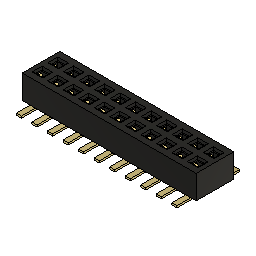
BD050-22-A-0-0500 (Autodesk Fusion 360 design; units mm, degrees)
Autodesk Fusion 360 part; units mm, degrees
note: some values were not read from the file. Chosen so that the rebuilt part matches the saved one: which bodies a step acts on. Set by a fixed rule: which sketch regions a step uses.
(part 1 of 3)
sketch "Sketch5" plane through (0, 0, 0) normal (0, 0, 1) x (1, 0, 0)
  line L0 (28.1987, -12.5621) -> (28.6114, -12.1494)
  line L1 (27.0768, -12.5992) -> (27.3573, -12.3134)
  line L2 (26.7911, -12.5198) -> (27.0768, -12.234)
  line L3 (27.4684, -11.853) -> (27.9817, -11.853)
  line L4 (27.3573, -11.9589) -> (28.1987, -11.9589)
  line L5 (26.68, -11.906) -> (26.8334, -11.7525)
  line L6 (26.8334, -11.7525) -> (26.68, -11.853)
  line L7 (26.68, -11.853) -> (26.68, -11.9589)
  line L8 (27.0768, -12.234) -> (27.4631, -11.8478)
  line L9 (27.0768, -11.8742) -> (27.1985, -11.7525)
  line L10 (27.4684, -11.9589) -> (27.4684, -11.853)
  line L11 (27.4684, -11.853) -> (27.315, -11.7525)
  line L12 (26.7911, -12.1547) -> (27.0768, -11.8742)
  line L13 (28.1987, -12.2023) -> (28.6114, -11.7843)
  line L14 (27.9817, -11.853) -> (27.9817, -11.9589)
  line L15 (28.077, -11.9589) -> (28.2833, -11.7525)
  line L16 (27.9817, -11.853) -> (28.1352, -11.7525)
  line L17 (25.537, -12.6838) -> (25.955, -12.2711)
  line L18 (25.537, -11.9589) -> (25.7486, -11.7525)
  line L19 (25.537, -12.324) -> (26.0714, -11.7895)
  line L20 (26.1667, -11.9589) -> (26.1667, -11.853)
  line L21 (26.1667, -11.853) -> (26.0132, -11.7525)
  line L22 (25.537, -11.7525) -> (28.6114, -11.7525)
  line L23 (26.7911, -11.9589) -> (25.955, -11.9589)
  line L24 (26.68, -11.853) -> (26.1667, -11.853)
  line L25 (27.0768, -13.684) -> (27.3573, -13.4035)
  line L26 (26.7911, -13.6046) -> (27.0768, -13.3241)
  line L27 (27.061, -13.6998) -> (27.0768, -13.684)
  line L28 (27.0768, -13.3241) -> (27.3573, -13.0384)
  line L29 (26.7911, -13.2395) -> (27.0768, -12.959)
  line L30 (28.1987, -13.6469) -> (28.6114, -13.2342)
  line L31 (28.6114, -13.8004) -> (28.3098, -13.8004)
  line L32 (28.3098, -13.8004) -> (28.1987, -13.6998)
  line L33 (28.405, -13.8004) -> (28.6114, -13.594)
  line L34 (28.1987, -13.2871) -> (28.6114, -12.8743)
  line L35 (25.537, -13.4088) -> (25.955, -12.996)
  line L36 (25.537, -13.7739) -> (25.955, -13.3559)
  line L37 (25.537, -13.8004) -> (25.8386, -13.8004)
  line L38 (25.8386, -13.8004) -> (25.955, -13.6998)
  line L39 (25.955, -13.6998) -> (28.1987, -13.6998)
  line L40 (28.1987, -13.6998) -> (28.1987, -11.9589)
  line L41 (28.6114, -11.7525) -> (28.6114, -13.8004)
  line L42 (27.3573, -11.9589) -> (27.3573, -13.6998)
  line L43 (26.7911, -11.9589) -> (26.7911, -13.6998)
  line L44 (25.955, -11.9589) -> (25.955, -13.6998)
  line L45 (27.8759, -12.16) -> (27.8706, -12.1335)
  line L46 (27.8706, -12.1335) -> (27.86, -12.107)
  line L47 (27.86, -12.107) -> (27.8441, -12.0912)
  line L48 (27.8441, -12.0912) -> (27.823, -12.0753)
  line L49 (27.823, -12.0753) -> (27.8018, -12.0647)
  line L50 (27.8018, -12.0647) -> (27.7753, -12.0594)
  line L51 (27.7753, -12.0594) -> (27.5795, -12.0594)
  line L52 (27.5795, -12.0594) -> (27.5531, -12.0647)
  line L53 (27.5531, -12.0647) -> (27.5266, -12.0753)
  line L54 (27.5266, -12.0753) -> (27.4949, -12.107)
  line L55 (27.4949, -12.107) -> (27.4843, -12.1335)
  line L56 (27.4843, -12.1335) -> (27.479, -12.16)
  line L57 (27.479, -12.16) -> (27.479, -13.086)
  line L58 (27.479, -13.086) -> (27.3255, -13.2871)
  line L59 (27.3255, -13.2871) -> (27.389, -13.2871)
  line L60 (27.4472, -13.3506) -> (27.442, -13.3294)
  line L61 (27.442, -13.3294) -> (27.4314, -13.3082)
  line L62 (27.4314, -13.3082) -> (27.4102, -13.2977)
  line L63 (27.4102, -13.2977) -> (27.389, -13.2924)
  line L64 (27.4472, -13.3506) -> (27.4472, -13.4935)
  line L65 (27.4525, -13.4935) -> (27.4578, -13.5199)
  line L66 (27.4578, -13.5199) -> (27.4684, -13.5411)
  line L67 (27.4684, -13.5411) -> (27.4843, -13.5623)
  line L68 (27.4843, -13.5623) -> (27.5002, -13.5781)
  line L69 (27.5002, -13.5781) -> (27.5266, -13.5887)
  line L70 (27.5266, -13.5887) -> (27.5531, -13.594)
  line L71 (27.5531, -13.594) -> (28.0452, -13.594)
  line L72 (28.0452, -13.594) -> (28.0452, -13.721)
  line L73 (28.0452, -13.721) -> (28.0505, -13.7686)
  line L74 (28.0505, -13.7686) -> (28.0611, -13.811)
  line L75 (28.0611, -13.811) -> (28.0822, -13.848)
  line L76 (28.0822, -13.848) -> (28.114, -13.885)
  line L77 (28.114, -13.885) -> (28.151, -13.9168)
  line L78 (28.151, -13.9168) -> (28.1881, -13.938)
  line L79 (28.1881, -13.938) -> (28.2304, -13.9485)
  line L80 (28.2304, -13.9485) -> (28.278, -13.9538)
  line L81 (28.278, -13.9538) -> (29.638, -13.9538)
  line L82 (29.638, -13.9538) -> (29.638, -13.8004)
  line L83 (29.638, -13.8004) -> (28.278, -13.8004)
  line L84 (28.1987, -13.721) -> (28.204, -13.7422)
  line L85 (28.204, -13.7422) -> (28.2092, -13.758)
  line L86 (28.2092, -13.758) -> (28.2198, -13.7792)
  line L87 (28.2198, -13.7792) -> (28.2357, -13.7898)
  line L88 (28.2357, -13.7898) -> (28.278, -13.8004)
  line L89 (28.1987, -13.721) -> (28.1987, -12.8796)
  line L90 (28.1987, -12.8796) -> (27.9817, -12.8796)
  line L91 (27.8812, -12.7738) -> (27.8865, -12.8002)
  line L92 (27.8865, -12.8002) -> (27.897, -12.8214)
  line L93 (27.897, -12.8214) -> (27.9129, -12.8426)
  line L94 (27.9129, -12.8426) -> (27.9288, -12.8585)
  line L95 (27.9288, -12.8585) -> (27.9552, -12.869)
  line L96 (27.9552, -12.869) -> (27.9817, -12.8743)
  line L97 (27.8812, -12.7738) -> (27.8812, -12.16)
  line L98 (25.537, -11.7525) -> (25.537, -13.8004)
  line L99 (26.373, -12.0594) -> (26.3466, -12.0647)
  line L100 (26.3466, -12.0647) -> (26.3201, -12.0753)
  line L101 (26.3201, -12.0753) -> (26.2884, -12.107)
  line L102 (26.2884, -12.107) -> (26.2778, -12.1335)
  line L103 (26.2778, -12.1335) -> (26.2725, -12.16)
  line L104 (26.373, -12.0594) -> (26.5688, -12.0594)
  line L105 (26.6694, -12.16) -> (26.6641, -12.1335)
  line L106 (26.6641, -12.1335) -> (26.6535, -12.107)
  line L107 (26.6535, -12.107) -> (26.6376, -12.0912)
  line L108 (26.6376, -12.0912) -> (26.6165, -12.0753)
  line L109 (26.6165, -12.0753) -> (26.5953, -12.0647)
  line L110 (26.5953, -12.0647) -> (26.5688, -12.0594)
  line L111 (26.6694, -12.16) -> (26.6694, -13.086)
  line L112 (26.6694, -13.086) -> (26.8281, -13.2871)
  line L113 (26.8281, -13.2871) -> (26.7646, -13.2871)
  line L114 (26.7646, -13.2924) -> (26.7435, -13.2977)
  line L115 (26.7435, -13.2977) -> (26.7223, -13.3083)
  line L116 (26.7223, -13.3083) -> (26.7117, -13.3294)
  line L117 (26.7117, -13.3294) -> (26.7064, -13.3506)
  line L118 (26.7011, -13.3506) -> (26.7011, -13.4935)
  line L119 (26.6006, -13.594) -> (26.627, -13.5887)
  line L120 (26.627, -13.5887) -> (26.6535, -13.5781)
  line L121 (26.6535, -13.5781) -> (26.6694, -13.5622)
  line L122 (26.6694, -13.5622) -> (26.6852, -13.5411)
  line L123 (26.6852, -13.5411) -> (26.6958, -13.5199)
  line L124 (26.6958, -13.5199) -> (26.7011, -13.4935)
  line L125 (26.6006, -13.594) -> (26.1085, -13.594)
  line L126 (26.1085, -13.594) -> (26.1085, -13.721)
  line L127 (25.8703, -13.9538) -> (25.918, -13.9485)
  line L128 (25.918, -13.9485) -> (25.9603, -13.938)
  line L129 (25.9603, -13.938) -> (25.9973, -13.9168)
  line L130 (25.9973, -13.9168) -> (26.0344, -13.885)
  line L131 (26.0344, -13.885) -> (26.0661, -13.848)
  line L132 (26.0661, -13.848) -> (26.0873, -13.811)
  line L133 (26.0873, -13.811) -> (26.0979, -13.7686)
  line L134 (26.0979, -13.7686) -> (26.1032, -13.721)
  line L135 (25.8703, -13.9538) -> (24.5104, -13.9538)
  line L136 (24.5104, -13.9538) -> (24.5104, -13.8004)
  line L137 (24.5104, -13.8004) -> (25.8703, -13.8004)
  line L138 (25.8703, -13.8004) -> (25.8915, -13.7951)
  line L139 (25.8915, -13.7951) -> (25.9074, -13.7898)
  line L140 (25.9074, -13.7898) -> (25.9285, -13.7792)
  line L141 (25.9285, -13.7792) -> (25.9391, -13.758)
  line L142 (25.9391, -13.758) -> (25.9444, -13.7422)
  line L143 (25.9444, -13.7422) -> (25.9497, -13.721)
  line L144 (25.955, -13.721) -> (25.955, -12.8796)
  line L145 (25.955, -12.8796) -> (26.1667, -12.8796)
  line L146 (26.1667, -12.8743) -> (26.1931, -12.869)
  line L147 (26.1931, -12.869) -> (26.2143, -12.8585)
  line L148 (26.2143, -12.8585) -> (26.2355, -12.8426)
  line L149 (26.2355, -12.8426) -> (26.2513, -12.8267)
  line L150 (26.2513, -12.8267) -> (26.2619, -12.8002)
  line L151 (26.2619, -12.8002) -> (26.2672, -12.7738)
  line L152 (26.2725, -12.7738) -> (26.2725, -12.16)
  line L153 (27.0768, -11.4615) -> (27.0768, -12.832)
  line L154 (27.0768, -13.086) -> (27.0768, -13.3453)
  line L155 (27.0768, -13.5993) -> (27.0768, -14.9698)
  line L156 (25.537, -13.049) -> (25.955, -12.6309)
  line L157 (27.0768, -12.959) -> (27.3573, -12.6785)
  line L158 (26.7911, -12.8796) -> (27.0768, -12.5992)
  line L159 (28.1987, -12.9272) -> (28.6114, -12.5092)
  line L160 (13.165, 1.9) -> (12.8581, 1.9)
  line L161 (14.4668, 1.9) -> (14.1599, 1.9)
  line L162 (14.5991, -0.296) -> (14.5991, 0.2702)
  line L163 (14.5991, 0.2702) -> (14.7261, 0.3972)
  line L164 (12.7311, 0.2702) -> (12.7311, -0.296)
  line L165 (11.9956, 0.2702) -> (11.9956, -0.296)
  line L166 (13.2973, 0.2702) -> (13.2973, -0.296)
  line L167 (13.2973, -0.296) -> (12.7311, -0.296)
  line L168 (11.9956, 0.2702) -> (12.1226, 0.3972)
  line L169 (13.4243, 0.3972) -> (13.2973, 0.2702)
  line L170 (13.2973, 0.2702) -> (12.7311, 0.2702)
  line L171 (12.7311, 0.2702) -> (12.6041, 0.3972)
  line L172 (12.6041, 0.3972) -> (13.4243, 0.3972)
  line L173 (14.0329, -0.296) -> (14.0329, 0.2702)
  line L174 (14.0329, 0.2702) -> (13.9059, 0.3972)
  line L175 (14.5991, -0.296) -> (14.0329, -0.296)
  line L176 (14.7261, 0.3972) -> (13.9059, 0.3972)
  line L177 (14.5991, 0.2702) -> (14.0329, 0.2702)
  line L178 (11.8686, 0.8734) -> (11.8686, 1.9)
  line L179 (13.165, 0.8734) -> (13.165, 1.9)
  line L180 (12.8581, 0.8734) -> (12.8581, 1.9)
  line L181 (14.4668, 0.8734) -> (14.4668, 1.9)
  line L182 (14.1599, 0.8734) -> (14.1599, 1.9)
  line L183 (10.5668, 1.9) -> (10.2546, 1.9)
  line L184 (7.9633, 1.9) -> (7.6564, 1.9)
  line L185 (7.6564, 1.9) -> (7.6564, 0.8734)
  line L186 (7.9633, 0.8734) -> (7.9633, 1.9)
  line L187 (9.2651, 0.8734) -> (9.2651, 1.9)
  line L188 (8.9582, 0.8734) -> (8.9582, 1.9)
  line L189 (8.9582, 1.9) -> (9.2651, 1.9)
  line L190 (10.6938, 0.2702) -> (10.6938, -0.296)
  line L191 (10.1276, 0.2702) -> (10.1276, -0.296)
  line L192 (11.4294, 0.2702) -> (11.4294, -0.296)
  line L193 (10.6938, -0.296) -> (10.1276, -0.296)
  line L194 (10.1276, 0.2702) -> (10.0006, 0.3972)
  line L195 (10.0006, 0.3972) -> (10.8208, 0.3972)
  line L196 (10.8208, 0.3972) -> (10.6938, 0.2702)
  line L197 (10.6938, 0.2702) -> (10.1276, 0.2702)
  line L198 (11.4294, 0.2702) -> (11.3024, 0.3972)
  line L199 (10.2546, 0.8734) -> (10.2546, 1.9)
  line L200 (10.5668, 0.8734) -> (10.5668, 1.9)
  line L201 (11.5564, 0.8734) -> (11.5564, 1.9)
  line L202 (-0.8367, 0.8734) -> (15.1494, 0.8734)
  line L203 (11.9956, -0.296) -> (11.4294, -0.296)
  line L204 (11.9956, 0.2702) -> (11.4294, 0.2702)
  line L205 (12.1226, 0.3972) -> (11.3024, 0.3972)
  line L206 (11.8686, 1.9) -> (11.5564, 1.9)
  line L207 (14.5991, -1.0316) -> (14.7261, -0.9046)
  line L208 (11.9956, -1.0316) -> (12.1226, -0.9046)
  line L209 (12.7311, -1.0316) -> (13.2973, -1.0316)
  line L210 (13.2973, -1.0316) -> (13.4243, -0.9046)
  line L211 (13.4243, -0.9046) -> (12.6041, -0.9046)
  line L212 (13.4243, -0.423) -> (12.6041, -0.423)
  line L213 (12.7311, -1.0316) -> (12.6041, -0.9046)
  line L214 (14.0329, -1.0316) -> (13.9059, -0.9046)
  line L215 (13.9059, -0.9046) -> (14.7261, -0.9046)
  line L216 (14.7261, -0.423) -> (13.9059, -0.423)
  line L217 (14.5991, -1.0316) -> (14.0329, -1.0316)
  line L218 (14.5991, -1.5978) -> (14.7261, -1.7248)
  line L219 (11.9956, -1.5978) -> (12.1226, -1.7248)
  line L220 (12.7311, -1.5978) -> (13.2973, -1.5978)
  line L221 (13.2973, -1.5978) -> (13.4243, -1.7248)
  line L222 (13.4243, -1.7248) -> (12.6041, -1.7248)
  line L223 (12.6041, -1.7248) -> (12.7311, -1.5978)
  line L224 (14.0329, -1.5978) -> (13.9059, -1.7248)
  line L225 (13.9059, -1.7248) -> (14.7261, -1.7248)
  line L226 (14.5991, -1.5978) -> (14.0329, -1.5978)
  line L227 (13.2973, -1.5978) -> (13.2973, -1.0316)
  line L228 (13.4243, -1.7248) -> (13.4243, -0.9046)
  line L229 (12.6041, -1.7248) -> (12.6041, -0.9046)
  line L230 (11.9956, -1.5978) -> (11.9956, -1.0316)
  line L231 (12.1226, -1.7248) -> (12.1226, -0.9046)
  line L232 (12.7311, -1.5978) -> (12.7311, -1.0316)
  line L233 (14.5991, -1.5978) -> (14.5991, -1.0316)
  line L234 (14.0329, -1.5978) -> (14.0329, -1.0316)
  line L235 (13.9059, -1.7248) -> (13.9059, -0.9046)
  line L236 (14.7261, -1.7248) -> (14.7261, -0.9046)
  line L237 (10.1276, -1.0316) -> (10.0006, -0.9046)
  line L238 (10.0006, -0.9046) -> (10.8208, -0.9046)
  line L239 (10.8208, -0.423) -> (10.0006, -0.423)
  line L240 (10.8208, -0.9046) -> (10.6938, -1.0316)
  line L241 (10.6938, -1.0316) -> (10.1276, -1.0316)
  line L242 (11.4294, -1.0316) -> (11.3024, -0.9046)
  line L243 (10.1276, -1.5978) -> (10.0006, -1.7248)
  line L244 (10.0006, -1.7248) -> (10.8208, -1.7248)
  line L245 (10.8208, -1.7248) -> (10.6938, -1.5978)
  line L246 (10.6938, -1.5978) -> (10.1276, -1.5978)
  line L247 (11.4294, -1.5978) -> (11.3024, -1.7248)
  line L248 (10.6938, -1.5978) -> (10.6938, -1.0316)
  line L249 (10.8208, -1.7248) -> (10.8208, -0.9046)
  line L250 (10.1276, -1.5978) -> (10.1276, -1.0316)
  line L251 (10.0006, -1.7248) -> (10.0006, -0.9046)
  line L252 (11.4294, -1.5978) -> (11.4294, -1.0316)
  line L253 (11.3024, -1.7248) -> (11.3024, -0.9046)
  line L254 (-0.8367, -2.201) -> (15.1494, -2.201)
  line L255 (11.9956, -1.5978) -> (11.4294, -1.5978)
  line L256 (12.1226, -1.7248) -> (11.3024, -1.7248)
  line L257 (11.9956, -1.0316) -> (11.4294, -1.0316)
  line L258 (12.1226, -0.9046) -> (11.3024, -0.9046)
  line L259 (12.1226, -0.423) -> (11.3024, -0.423)
  line L260 (10.8208, 0.3972) -> (10.8208, -0.423)
  line L261 (10.0006, 0.3972) -> (10.0006, -0.423)
  line L262 (11.3024, 0.3972) -> (11.3024, -0.423)
  line L263 (12.6041, 0.3972) -> (12.6041, -0.423)
  line L264 (12.1226, 0.3972) -> (12.1226, -0.423)
  line L265 (13.4243, 0.3972) -> (13.4243, -0.423)
  line L266 (10.1276, -0.296) -> (10.0006, -0.423)
  line L267 (10.6938, -0.296) -> (10.8208, -0.423)
  line L268 (11.9956, -0.296) -> (12.1226, -0.423)
  line L269 (11.4294, -0.296) -> (11.3024, -0.423)
  line L270 (13.2973, -0.296) -> (13.4243, -0.423)
  line L271 (12.7311, -0.296) -> (12.6041, -0.423)
  line L272 (13.9059, 0.3972) -> (13.9059, -0.423)
  line L273 (15.1494, -2.201) -> (15.1494, 0.8734)
  line L274 (15.1494, 0.8734) -> (15.1494, -2.201)
  line L275 (14.7261, 0.3972) -> (14.7261, -0.423)
  line L276 (14.7261, -0.423) -> (14.5991, -0.296)
  line L277 (14.0329, -0.296) -> (13.9059, -0.423)
  line L278 (6.6616, 1.9) -> (6.3547, 1.9)
  line L279 (5.0529, 1.9) -> (5.3598, 1.9)
  line L280 (5.3598, 1.9) -> (5.3598, 0.8734)
  line L281 (5.0529, 0.8734) -> (5.0529, 1.9)
  line L282 (6.3547, 0.8734) -> (6.3547, 1.9)
  line L283 (6.6616, 0.8734) -> (6.6616, 1.9)
  line L284 (2.7563, 1.9) -> (2.4494, 1.9)
  line L285 (4.0581, 1.9) -> (3.7512, 1.9)
  line L286 (3.4919, 0.3972) -> (4.3121, 0.3972)
  line L287 (4.3121, 0.3972) -> (4.1851, 0.2702)
  line L288 (2.8833, 0.2702) -> (2.8833, -0.296)
  line L289 (2.3224, 0.2702) -> (2.3224, -0.296)
  line L290 (3.6242, 0.2702) -> (3.6242, -0.296)
  line L291 (4.1851, 0.2702) -> (4.1851, -0.296)
  line L292 (2.3224, -0.296) -> (2.8833, -0.296)
  line L293 (3.6242, -0.296) -> (4.1851, -0.296)
  line L294 (2.8833, 0.2702) -> (3.0103, 0.3972)
  line L295 (2.1901, 0.3972) -> (2.3224, 0.2702)
  line L296 (2.3224, 0.2702) -> (2.8833, 0.2702)
  line L297 (2.1901, 0.3972) -> (3.0103, 0.3972)
  line L298 (3.4919, 0.3972) -> (3.6242, 0.2702)
  line L299 (3.6242, 0.2702) -> (4.1851, 0.2702)
  line L300 (2.7563, 0.8734) -> (2.7563, 1.9)
  line L301 (2.4494, 0.8734) -> (2.4494, 1.9)
  line L302 (3.7512, 0.8734) -> (3.7512, 1.9)
  line L303 (4.0581, 0.8734) -> (4.0581, 1.9)
  line L304 (0.1528, 1.9) -> (-0.1541, 1.9)
  line L305 (1.4546, 1.9) -> (1.1477, 1.9)
  line L306 (1.5816, 0.2702) -> (1.5816, -0.296)
  line L307 (0.2798, 0.2702) -> (0.2798, -0.296)
  line L308 (1.0207, 0.2702) -> (1.0207, -0.296)
  line L309 (1.0207, -0.296) -> (1.5816, -0.296)
  line L310 (0.2798, 0.2702) -> (0.4121, 0.3972)
  line L311 (1.7086, 0.3972) -> (1.5816, 0.2702)
  line L312 (1.5816, 0.2702) -> (1.0207, 0.2702)
  line L313 (1.0207, 0.2702) -> (0.8937, 0.3972)
  line L314 (0.8937, 0.3972) -> (1.7086, 0.3972)
  line L315 (-0.2811, -0.296) -> (-0.2811, 0.2702)
  line L316 (-0.2811, 0.2702) -> (-0.4081, 0.3972)
  line L317 (-0.2811, -0.296) -> (0.2798, -0.296)
  line L318 (-0.4081, 0.3972) -> (0.4121, 0.3972)
  line L319 (-0.2811, 0.2702) -> (0.2798, 0.2702)
  line L320 (1.4546, 0.8734) -> (1.4546, 1.9)
  line L321 (0.1528, 0.8734) -> (0.1528, 1.9)
  line L322 (-0.1541, 0.8734) -> (-0.1541, 1.9)
  line L323 (1.1477, 0.8734) -> (1.1477, 1.9)
  line L324 (3.4919, -0.9046) -> (4.3121, -0.9046)
  line L325 (3.4919, -0.423) -> (4.3121, -0.423)
  line L326 (4.1851, -1.0316) -> (4.3121, -0.9046)
  line L327 (2.8833, -1.0316) -> (3.0103, -0.9046)
  line L328 (2.3224, -1.0316) -> (2.1901, -0.9046)
  line L329 (2.1901, -0.9046) -> (3.0103, -0.9046)
  line L330 (2.3224, -1.0316) -> (2.8833, -1.0316)
  line L331 (2.1901, -0.423) -> (3.0103, -0.423)
  line L332 (3.4919, -0.9046) -> (3.6242, -1.0316)
  line L333 (3.6242, -1.0316) -> (4.1851, -1.0316)
  line L334 (3.4919, -1.7248) -> (4.3121, -1.7248)
  line L335 (4.3121, -1.7248) -> (4.1851, -1.5978)
  line L336 (2.8833, -1.5978) -> (3.0103, -1.7248)
  line L337 (2.3224, -1.5978) -> (2.1901, -1.7248)
  line L338 (2.1901, -1.7248) -> (3.0103, -1.7248)
  line L339 (2.3224, -1.5978) -> (2.8833, -1.5978)
  line L340 (3.4919, -1.7248) -> (3.6242, -1.5978)
  line L341 (3.6242, -1.5978) -> (4.1851, -1.5978)
  line L342 (3.4919, -1.7248) -> (3.4919, -0.9046)
  line L343 (3.6242, -1.5978) -> (3.6242, -1.0316)
  line L344 (3.0103, -1.7248) -> (3.0103, -0.9046)
  line L345 (2.8833, -1.5978) -> (2.8833, -1.0316)
  line L346 (2.1901, -1.7248) -> (2.1901, -0.9046)
  line L347 (2.3224, -1.5978) -> (2.3224, -1.0316)
  line L348 (4.1851, -1.5978) -> (4.1851, -1.0316)
  line L349 (4.3121, -1.7248) -> (4.3121, -0.9046)
  line L350 (0.2798, -1.0316) -> (0.4121, -0.9046)
  line L351 (1.7086, -0.9046) -> (1.5816, -1.0316)
  line L352 (1.5816, -1.0316) -> (1.0207, -1.0316)
  line L353 (0.8937, -0.423) -> (1.7086, -0.423)
  line L354 (1.7086, -0.9046) -> (0.8937, -0.9046)
  line L355 (0.8937, -0.9046) -> (1.0207, -1.0316)
  line L356 (-0.2811, -1.0316) -> (-0.4081, -0.9046)
  line L357 (-0.4081, -0.9046) -> (0.4121, -0.9046)
  line L358 (-0.2811, -1.0316) -> (0.2798, -1.0316)
  line L359 (-0.4081, -0.423) -> (0.4121, -0.423)
  line L360 (0.2798, -1.5978) -> (0.4121, -1.7248)
  line L361 (1.7086, -1.7248) -> (1.5816, -1.5978)
  line L362 (1.5816, -1.5978) -> (1.0207, -1.5978)
  line L363 (1.7086, -1.7248) -> (0.8937, -1.7248)
  line L364 (0.8937, -1.7248) -> (1.0207, -1.5978)
  line L365 (-0.2811, -1.5978) -> (-0.4081, -1.7248)
  line L366 (-0.4081, -1.7248) -> (0.4121, -1.7248)
  line L367 (-0.2811, -1.5978) -> (0.2798, -1.5978)
  line L368 (0.2798, -1.5978) -> (0.2798, -1.0316)
  line L369 (0.4121, -1.7248) -> (0.4121, -0.9046)
  line L370 (1.0207, -1.5978) -> (1.0207, -1.0316)
  line L371 (0.8937, -1.7248) -> (0.8937, -0.9046)
  line L372 (1.7086, -1.7248) -> (1.7086, -0.9046)
  line L373 (1.5816, -1.5978) -> (1.5816, -1.0316)
  line L374 (-0.4081, -1.7248) -> (-0.4081, -0.9046)
  line L375 (-0.2811, -1.5978) -> (-0.2811, -1.0316)
  line L376 (-0.8367, 0.8734) -> (-0.8367, -2.201)
  line L377 (4.1851, -0.296) -> (4.3121, -0.423)
  line L378 (3.4919, 0.3972) -> (3.4919, -0.423)
  line L379 (0.4121, 0.3972) -> (0.4121, -0.423)
  line L380 (0.8937, 0.3972) -> (0.8937, -0.423)
  line L381 (3.0103, 0.3972) -> (3.0103, -0.423)
  line L382 (2.1901, 0.3972) -> (2.1901, -0.423)
  line L383 (1.7086, 0.3972) -> (1.7086, -0.423)
  line L384 (-0.4081, 0.3972) -> (-0.4081, -0.423)
  line L385 (0.2798, -0.296) -> (0.4121, -0.423)
  line L386 (-0.2811, -0.296) -> (-0.4081, -0.423)
  line L387 (1.5816, -0.296) -> (1.7086, -0.423)
  line L388 (1.0207, -0.296) -> (0.8937, -0.423)
  line L389 (2.8833, -0.296) -> (3.0103, -0.423)
  line L390 (2.3224, -0.296) -> (2.1901, -0.423)
  line L391 (3.6242, -0.296) -> (3.4919, -0.423)
  line L392 (4.3121, 0.3972) -> (4.3121, -0.423)
  line L393 (13.165, -3.2276) -> (12.8581, -3.2276)
  line L394 (14.4668, -3.2276) -> (14.1599, -3.2276)
  line L395 (10.5668, -3.2276) -> (10.2546, -3.2276)
  line L396 (7.9633, -3.2276) -> (7.6564, -3.2276)
  line L397 (9.2651, -3.2276) -> (8.9582, -3.2276)
  line L398 (11.8686, -3.2276) -> (11.5564, -3.2276)
  line L399 (14.7261, -11.7525) -> (14.5991, -11.853)
  line L400 (14.5991, -11.853) -> (14.5991, -11.9589)
  line L401 (13.5831, -11.7525) -> (13.6678, -12.287)
  line L402 (13.9059, -11.7525) -> (14.0329, -11.853)
  line L403 (14.0329, -11.853) -> (14.0329, -11.9589)
  line L404 (13.8159, -11.9589) -> (14.8108, -11.9589)
  line L405 (14.0329, -11.853) -> (14.5991, -11.853)
  line L406 (-0.8367, -11.7525) -> (15.1494, -11.7525)
  line L407 (14.5303, -13.594) -> (14.7843, -13.594)
  line L408 (14.5303, -13.8004) -> (15.1494, -13.8004)
  line L409 (14.5303, -13.6998) -> (15.1494, -13.6998)
  line L410 (14.5303, -13.594) -> (14.5303, -13.9538)
  line L411 (14.6308, -13.0331) -> (14.7843, -13.0331)
  line L412 (13.5249, -13.2712) -> (13.6625, -13.8004)
  line L413 (11.9268, -13.9538) -> (11.9268, -13.8004)
  line L414 (12.7999, -13.9538) -> (13.2285, -13.9538)
  line L415 (13.2285, -13.8004) -> (12.7999, -13.8004)
  line L416 (12.7999, -13.8004) -> (12.7999, -13.9538)
  line L417 (13.2285, -13.9538) -> (13.2285, -13.8004)
  line L418 (14.1017, -13.9538) -> (14.1017, -13.594)
  line L419 (14.1017, -13.594) -> (13.8424, -13.594)
  line L420 (13.636, -13.6998) -> (14.1017, -13.6998)
  line L421 (13.8424, -13.0331) -> (13.9958, -13.0331)
  line L422 (14.5303, -13.9538) -> (14.1017, -13.9538)
  line L423 (14.5303, -13.8004) -> (14.1017, -13.8004)
  line L424 (13.9958, -12.8796) -> (14.6308, -12.8796)
  line L425 (10.625, -13.9538) -> (10.625, -13.8004)
  line L426 (10.1964, -13.9538) -> (10.1964, -13.8004)
  line L427 (10.1964, -13.8004) -> (10.625, -13.8004)
  line L428 (10.1964, -13.9538) -> (10.625, -13.9538)
  line L429 (11.4982, -13.8004) -> (11.4982, -13.9538)
  line L430 (8.8947, -13.8004) -> (9.3233, -13.8004)
  line L431 (8.8947, -13.9538) -> (9.3233, -13.9538)
  line L432 (7.5929, -13.8004) -> (8.0215, -13.8004)
  line L433 (8.0215, -13.9538) -> (7.5929, -13.9538)
  line L434 (7.5929, -13.9538) -> (7.5929, -13.8004)
  line L435 (8.8947, -13.8004) -> (8.8947, -13.9538)
  line L436 (8.0215, -13.9538) -> (8.0215, -13.8004)
  line L437 (9.3233, -13.9538) -> (9.3233, -13.8004)
  line L438 (11.4982, -13.9538) -> (11.9268, -13.9538)
  line L439 (11.4982, -13.8004) -> (11.9268, -13.8004)
  line L440 (7.159, -11.3715) -> (7.159, -12.3981)
  line L441 (7.159, -12.6521) -> (7.159, -12.9114)
  line L442 (7.159, -13.1654) -> (7.159, -14.192)
  line L443 (14.7843, -13.594) -> (14.7843, -12.795)
  line L444 (14.7843, -12.795) -> (14.7843, -12.7579)
  line L445 (14.7843, -12.7579) -> (14.7737, -12.7156)
  line L446 (14.779, -12.7209) -> (14.6467, -12.4034)
  line L447 (14.652, -12.3134) -> (14.6467, -12.3346)
  line L448 (14.6467, -12.3346) -> (14.6414, -12.361)
  line L449 (14.6414, -12.361) -> (14.6414, -12.3822)
  line L450 (14.6414, -12.3822) -> (14.6467, -12.4034)
  line L451 (14.652, -12.3134) -> (14.7367, -12.1123)
  line L452 (14.7367, -12.1123) -> (14.5938, -12.0594)
  line L453 (14.5938, -12.0594) -> (14.5091, -12.2605)
  line L454 (14.5038, -12.2605) -> (14.4933, -12.3081)
  line L455 (14.4933, -12.3081) -> (14.488, -12.3505)
  line L456 (14.488, -12.3505) -> (14.488, -12.3981)
  line L457 (14.488, -12.3981) -> (14.4985, -12.4457)
  line L458 (14.4985, -12.4457) -> (14.6255, -12.7579)
  line L459 (14.6308, -12.795) -> (14.6308, -12.7738)
  line L460 (14.6308, -12.7738) -> (14.6255, -12.7579)
  line L461 (14.6308, -12.795) -> (14.6308, -13.594)
  line L462 (13.8424, -13.594) -> (13.8424, -12.795)
  line L463 (13.853, -12.7156) -> (13.8424, -12.7579)
  line L464 (13.8424, -12.7579) -> (13.8424, -12.795)
  line L465 (13.853, -12.7209) -> (13.98, -12.4034)
  line L466 (13.98, -12.4034) -> (13.9853, -12.3822)
  line L467 (13.9853, -12.3822) -> (13.9853, -12.361)
  line L468 (13.9853, -12.361) -> (13.98, -12.3346)
  line L469 (13.98, -12.3346) -> (13.9747, -12.3134)
  line L470 (13.98, -12.3134) -> (13.8953, -12.1123)
  line L471 (13.8953, -12.1123) -> (14.0382, -12.0594)
  line L472 (14.0382, -12.0594) -> (14.1228, -12.2605)
  line L473 (14.1281, -12.4457) -> (14.1387, -12.3981)
  line L474 (14.1387, -12.3981) -> (14.1387, -12.3505)
  line L475 (14.1387, -12.3505) -> (14.1334, -12.3081)
  line L476 (14.1334, -12.3081) -> (14.1228, -12.2605)
  line L477 (14.1334, -12.4457) -> (14.0011, -12.7579)
  line L478 (14.0011, -12.7579) -> (13.9958, -12.7738)
  line L479 (13.9958, -12.7738) -> (13.9958, -12.795)
  line L480 (13.9958, -12.795) -> (13.9958, -13.594)
  line L481 (14.8108, -11.9589) -> (14.8107, -13.6998)
  line L482 (15.1494, -11.7525) -> (15.1494, -13.8004)
  line L483 (13.8159, -11.9589) -> (13.8159, -13.6998)
  line L484 (13.6678, -12.287) -> (13.5249, -13.2712)
  line L485 (13.5884, -11.7631) -> (13.599, -11.7525)
  line L486 (13.636, -12.0753) -> (13.9376, -11.779)
  line L487 (13.6466, -12.4298) -> (13.8159, -12.2605)
  line L488 (13.5831, -12.8532) -> (13.8159, -12.6203)
  line L489 (13.5249, -13.2765) -> (13.8159, -12.9802)
  line L490 (14.8107, -11.9906) -> (15.0489, -11.7525)
  line L491 (13.599, -13.5622) -> (13.8159, -13.3453)
  line L492 (14.8107, -12.3505) -> (15.1494, -12.0118)
  line L493 (14.8107, -12.7156) -> (15.1494, -12.3769)
  line L494 (14.8107, -13.0754) -> (15.1494, -12.7368)
  line L495 (14.8107, -13.4352) -> (15.1494, -13.1019)
  line L496 (14.9642, -13.6469) -> (15.1494, -13.4617)
  line L497 (6.6616, -3.2276) -> (6.3547, -3.2276)
  line L498 (5.3598, -3.2276) -> (5.0529, -3.2276)
  line L499 (2.7563, -3.2276) -> (2.4494, -3.2276)
  line L500 (4.0581, -3.2276) -> (3.7512, -3.2276)
  line L501 (0.1528, -3.2276) -> (-0.1541, -3.2276)
  line L502 (1.4546, -3.2276) -> (1.1477, -3.2276)
  line L503 (6.2912, -13.8004) -> (6.7198, -13.8004)
  line L504 (6.2912, -13.9538) -> (6.7198, -13.9538)
  line L505 (4.9894, -13.8004) -> (5.418, -13.8004)
  line L506 (5.418, -13.9538) -> (4.9894, -13.9538)
  line L507 (4.9894, -13.9538) -> (4.9894, -13.8004)
  line L508 (5.418, -13.9538) -> (5.418, -13.8004)
  line L509 (6.2912, -13.8004) -> (6.2912, -13.9538)
  line L510 (6.7198, -13.9538) -> (6.7198, -13.8004)
  line L511 (2.3859, -13.8004) -> (2.8198, -13.8004)
  line L512 (2.8198, -13.8004) -> (2.8198, -13.9538)
  line L513 (2.3859, -13.8004) -> (2.3859, -13.9538)
  line L514 (2.3859, -13.9538) -> (2.8198, -13.9538)
  line L515 (3.6877, -13.8004) -> (4.1216, -13.8004)
  line L516 (4.1216, -13.8004) -> (4.1216, -13.9538)
  line L517 (3.6877, -13.8004) -> (3.6877, -13.9538)
  line L518 (3.6877, -13.9538) -> (4.1216, -13.9538)
  line L519 (0.2163, -13.9538) -> (0.2163, -13.8004)
  line L520 (-0.2176, -13.8004) -> (-0.2176, -13.9538)
  line L521 (-0.2176, -13.9538) -> (0.2163, -13.9538)
  line L522 (-0.2176, -13.8004) -> (0.2163, -13.8004)
  line L523 (1.5181, -13.9538) -> (1.5181, -13.8004)
  line L524 (1.0842, -13.9538) -> (1.0842, -13.8004)
  line L525 (1.0842, -13.8004) -> (1.5181, -13.8004)
  line L526 (1.0842, -13.9538) -> (1.5181, -13.9538)
  line L527 (-0.8367, -13.8004) -> (-0.8367, -11.7525)
  line L528 (-0.8367, -13.6998) -> (13.636, -13.6998)
  line L529 (-0.8367, -13.8004) -> (14.1017, -13.8004)
  line L530 (14.4668, -2.201) -> (14.4668, -3.2276)
  line L531 (14.1599, -2.201) -> (14.1599, -3.2276)
  line L532 (10.2546, -2.201) -> (10.2546, -3.2276)
  line L533 (10.5668, -2.201) -> (10.5668, -3.2276)
  line L534 (9.2651, -2.201) -> (9.2651, -3.2276)
  line L535 (11.5564, -2.201) -> (11.5564, -3.2276)
  line L536 (13.165, -2.201) -> (13.165, -3.2276)
  line L537 (12.8581, -2.201) -> (12.8581, -3.2276)
  line L538 (11.8686, -2.201) -> (11.8686, -3.2276)
  line L539 (6.6616, -2.201) -> (6.6616, -3.2276)
  line L540 (6.3547, -2.201) -> (6.3547, -3.2276)
  line L541 (5.0529, -2.201) -> (5.0529, -3.2276)
  line L542 (5.3598, -2.201) -> (5.3598, -3.2276)
  line L543 (7.9633, -2.201) -> (7.9633, -3.2276)
  line L544 (7.6564, -2.201) -> (7.6564, -3.2276)
  line L545 (8.9582, -2.201) -> (8.9582, -3.2276)
  line L546 (-0.1541, -2.201) -> (-0.1541, -3.2276)
  line L547 (0.1528, -2.201) -> (0.1528, -3.2276)
  line L548 (2.7563, -2.201) -> (2.7563, -3.2276)
  line L549 (1.4546, -2.201) -> (1.4546, -3.2276)
  line L550 (1.1477, -2.201) -> (1.1477, -3.2276)
  line L551 (2.4494, -2.201) -> (2.4494, -3.2276)
  line L552 (3.7512, -2.201) -> (3.7512, -3.2276)
  line L553 (4.0581, -2.201) -> (4.0581, -3.2276)
  line L554 (14.488, -1.5978) -> (14.488, -1.0316)
  line L555 (14.1387, -1.5978) -> (14.1387, -1.0316)
  line L556 (14.1387, -0.296) -> (14.1387, 0.2702)
  line L557 (14.488, -0.296) -> (14.488, 0.2702)
  line L558 (12.837, -1.5978) -> (12.837, -1.0316)
  line L559 (13.1862, -1.5978) -> (13.1862, -1.0316)
  line L560 (13.1862, -0.296) -> (13.1862, 0.2702)
  line L561 (12.837, -0.296) -> (12.837, 0.2702)
  line L562 (11.5405, -1.5978) -> (11.5405, -1.0316)
  line L563 (11.8845, -1.5978) -> (11.8845, -1.0316)
  line L564 (11.8845, -0.296) -> (11.8845, 0.2702)
  line L565 (11.5405, -0.296) -> (11.5405, 0.2702)
  line L566 (10.2387, -1.5978) -> (10.2387, -1.0316)
  line L567 (10.5827, -1.5978) -> (10.5827, -1.0316)
  line L568 (10.5827, -0.296) -> (10.5827, 0.2702)
  line L569 (10.2387, -0.296) -> (10.2387, 0.2702)
  line L570 (3.73, -1.5978) -> (3.73, -1.0316)
  line L571 (4.0793, -1.5978) -> (4.0793, -1.0316)
  line L572 (4.0793, -0.296) -> (4.0793, 0.2702)
  line L573 (3.73, -0.296) -> (3.73, 0.2702)
  line L574 (2.4283, -1.5978) -> (2.4283, -1.0316)
  line L575 (2.7775, -1.5978) -> (2.7775, -1.0316)
  line L576 (2.7775, -0.296) -> (2.7775, 0.2702)
  line L577 (2.4283, -0.296) -> (2.4283, 0.2702)
  line L578 (1.1265, -1.5978) -> (1.1265, -1.0316)
  line L579 (1.4758, -1.5978) -> (1.4758, -1.0316)
  line L580 (1.4758, -0.296) -> (1.4758, 0.2702)
  line L581 (1.1265, -0.296) -> (1.1265, 0.2702)
  line L582 (-0.1752, -1.5978) -> (-0.1752, -1.0316)
  line L583 (0.174, -1.5978) -> (0.174, -1.0316)
  line L584 (0.174, -0.296) -> (0.174, 0.2702)
  line L585 (-0.1752, -0.296) -> (-0.1752, 0.2702)
  line L586 (9.2863, -0.296) -> (9.2863, 0.2702)
  line L587 (8.937, -0.296) -> (8.937, 0.2702)
  line L588 (8.937, -1.5978) -> (8.937, -1.0316)
  line L589 (9.2863, -1.5978) -> (9.2863, -1.0316)
  line L590 (7.9845, -0.296) -> (7.9845, 0.2702)
  line L591 (7.6352, -0.296) -> (7.6352, 0.2702)
  line L592 (7.6352, -1.5978) -> (7.6352, -1.0316)
  line L593 (7.9845, -1.5978) -> (7.9845, -1.0316)
  line L594 (6.3335, -0.296) -> (6.3335, 0.2702)
  line L595 (6.6827, -0.296) -> (6.6827, 0.2702)
  line L596 (6.6827, -1.5978) -> (6.6827, -1.0316)
  line L597 (6.3335, -1.5978) -> (6.3335, -1.0316)
  line L598 (6.7886, -0.296) -> (6.9156, -0.423)
  line L599 (6.2224, -0.296) -> (6.0954, -0.423)
  line L600 (6.0954, -0.423) -> (6.0954, 0.3972)
  line L601 (6.9156, 0.3972) -> (6.9156, -0.423)
  line L602 (8.0903, -0.296) -> (8.2173, -0.423)
  line L603 (7.5241, -0.296) -> (7.3971, -0.423)
  line L604 (9.3921, -0.296) -> (9.5191, -0.423)
  line L605 (8.8259, -0.296) -> (8.6989, -0.423)
  line L606 (7.3971, 0.3972) -> (7.3971, -0.423)
  line L607 (8.6989, 0.3972) -> (8.6989, -0.423)
  line L608 (8.2173, 0.3972) -> (8.2173, -0.423)
  line L609 (9.5191, 0.3972) -> (9.5191, -0.423)
  line L610 (9.5191, -0.423) -> (8.6989, -0.423)
  line L611 (8.6989, -0.9046) -> (9.5191, -0.9046)
  line L612 (8.8259, -1.0316) -> (9.3921, -1.0316)
  line L613 (8.6989, -1.7248) -> (9.5191, -1.7248)
  line L614 (8.8259, -1.5978) -> (9.3921, -1.5978)
  line L615 (9.5191, -1.7248) -> (9.5191, -0.9046)
  line L616 (9.3921, -1.0316) -> (9.3921, -1.5978)
  line L617 (9.3921, -1.5978) -> (9.5191, -1.7248)
  line L618 (9.3921, -1.0316) -> (9.5191, -0.9046)
  line L619 (6.0954, -1.7248) -> (6.0954, -0.9046)
  line L620 (6.9156, -1.7248) -> (6.9156, -0.9046)
  line L621 (6.7886, -1.5978) -> (6.7886, -1.0316)
  line L622 (6.2224, -1.5978) -> (6.2224, -1.0316)
  line L623 (8.0903, -1.5978) -> (8.0903, -1.0316)
  line L624 (8.6989, -1.7248) -> (8.6989, -0.9046)
  line L625 (8.8259, -1.5978) -> (8.8259, -1.0316)
  line L626 (8.2173, -1.7248) -> (8.2173, -0.9046)
  line L627 (7.3971, -1.7248) -> (7.3971, -0.9046)
  line L628 (7.5241, -1.5978) -> (7.5241, -1.0316)
  line L629 (6.2224, -1.5978) -> (6.7886, -1.5978)
  line L630 (6.0954, -1.7248) -> (6.9156, -1.7248)
  line L631 (6.9156, -1.7248) -> (6.7886, -1.5978)
  line L632 (8.0903, -1.5978) -> (8.2173, -1.7248)
  line L633 (8.2173, -1.7248) -> (7.3971, -1.7248)
  line L634 (7.3971, -1.7248) -> (7.5241, -1.5978)
  line L635 (7.5241, -1.5978) -> (8.0903, -1.5978)
  line L636 (8.8259, -1.5978) -> (8.6989, -1.7248)
  line L637 (6.2224, -1.5978) -> (6.0954, -1.7248)
  line L638 (6.2224, -1.0316) -> (6.7886, -1.0316)
  line L639 (6.0954, -0.423) -> (6.9156, -0.423)
  line L640 (6.0954, -0.9046) -> (6.9156, -0.9046)
  line L641 (6.9156, -0.9046) -> (6.7886, -1.0316)
  line L642 (8.0903, -1.0316) -> (8.2173, -0.9046)
  line L643 (7.3971, -0.423) -> (8.2173, -0.423)
  line L644 (8.2173, -0.9046) -> (7.3971, -0.9046)
  line L645 (7.3971, -0.9046) -> (7.5241, -1.0316)
  line L646 (7.5241, -1.0316) -> (8.0903, -1.0316)
  line L647 (8.8259, -1.0316) -> (8.6989, -0.9046)
  line L648 (6.2224, -1.0316) -> (6.0954, -0.9046)
  line L649 (8.6989, 0.3972) -> (9.5191, 0.3972)
  line L650 (8.8259, 0.2702) -> (9.3921, 0.2702)
  line L651 (8.8259, -0.296) -> (9.3921, -0.296)
  line L652 (9.5191, 0.3972) -> (9.3921, 0.2702)
  line L653 (9.3921, 0.2702) -> (9.3921, -0.296)
  line L654 (6.2224, 0.2702) -> (6.7886, 0.2702)
  line L655 (6.0954, 0.3972) -> (6.9156, 0.3972)
  line L656 (6.2224, -0.296) -> (6.7886, -0.296)
  line L657 (6.9156, 0.3972) -> (6.7886, 0.2702)
  line L658 (6.7886, 0.2702) -> (6.7886, -0.296)
  line L659 (7.3971, 0.3972) -> (8.2173, 0.3972)
  line L660 (8.2173, 0.3972) -> (8.0903, 0.2702)
  line L661 (8.0903, 0.2702) -> (7.5241, 0.2702)
  line L662 (7.5241, 0.2702) -> (7.3971, 0.3972)
  line L663 (8.8259, 0.2702) -> (8.6989, 0.3972)
  line L664 (8.0903, -0.296) -> (7.5241, -0.296)
  line L665 (7.5241, -0.296) -> (7.5241, 0.2702)
  line L666 (8.8259, 0.2702) -> (8.8259, -0.296)
  line L667 (8.0903, 0.2702) -> (8.0903, -0.296)
  line L668 (6.0954, 0.3972) -> (6.2224, 0.2702)
  line L669 (6.2224, 0.2702) -> (6.2224, -0.296)
  line L670 (4.9259, 0.2702) -> (4.9259, -0.296)
  line L671 (5.4868, 0.2702) -> (5.4868, -0.296)
  line L672 (5.4868, -0.296) -> (4.9259, -0.296)
  line L673 (5.6138, 0.3972) -> (5.4868, 0.2702)
  line L674 (5.4868, 0.2702) -> (4.9259, 0.2702)
  line L675 (4.9259, 0.2702) -> (4.7936, 0.3972)
  line L676 (4.7936, 0.3972) -> (5.6138, 0.3972)
  line L677 (4.9259, -1.0316) -> (5.4868, -1.0316)
  line L678 (5.4868, -1.0316) -> (5.6138, -0.9046)
  line L679 (5.6138, -0.9046) -> (4.7936, -0.9046)
  line L680 (5.6138, -0.423) -> (4.7936, -0.423)
  line L681 (4.9259, -1.0316) -> (4.7936, -0.9046)
  line L682 (4.9259, -1.5978) -> (5.4868, -1.5978)
  line L683 (5.4868, -1.5978) -> (5.6138, -1.7248)
  line L684 (5.6138, -1.7248) -> (4.7936, -1.7248)
  line L685 (4.7936, -1.7248) -> (4.9259, -1.5978)
  line L686 (5.4868, -1.5978) -> (5.4868, -1.0316)
  line L687 (5.6138, -1.7248) -> (5.6138, -0.9046)
  line L688 (4.7936, -1.7248) -> (4.7936, -0.9046)
  line L689 (4.9259, -1.5978) -> (4.9259, -1.0316)
  line L690 (4.7936, 0.3972) -> (4.7936, -0.423)
  line L691 (5.6138, 0.3972) -> (5.6138, -0.423)
  line L692 (5.6138, -0.423) -> (5.4868, -0.296)
  line L693 (4.9259, -0.296) -> (4.7936, -0.423)
  line L694 (5.0317, -1.5978) -> (5.0317, -1.0316)
  line L695 (5.381, -1.5978) -> (5.381, -1.0316)
  line L696 (5.381, -0.296) -> (5.381, 0.2702)
  line L697 (5.0317, -0.296) -> (5.0317, 0.2702)
  line L698 (-0.0006, -3.3917) -> (-0.0006, -6.191)
  line L699 (14.3133, -3.3917) -> (14.3133, -6.191)
  line L700 (0.5709, -6.0269) -> (13.7418, -6.0269)
  line L701 (0.5709, -5.9317) -> (0.5709, -6.1222)
  line L702 (0.5709, -6.1222) -> (-0.0006, -6.0269)
  line L703 (13.7418, -5.9317) -> (13.7418, -6.1222)
  line L704 (13.7418, -6.1222) -> (14.3133, -6.0269)
  line L705 (-0.8367, -2.3651) -> (-0.8367, -7.3234)
  line L706 (15.1494, -2.3651) -> (15.1494, -7.3234)
  line L707 (-0.2599, -7.1593) -> (14.5779, -7.1593)
  line L708 (-0.2599, -7.0641) -> (-0.2599, -7.2546)
  line L709 (-0.2599, -7.2546) -> (-0.8367, -7.1593)
  line L710 (14.5779, -7.0641) -> (14.5779, -7.2546)
  line L711 (14.5779, -7.2546) -> (15.1494, -7.1593)
  line L712 (14.7631, -1.312) -> (16.5835, -1.312)
  line L713 (14.7631, -0.0156) -> (16.5835, -0.0156)
  line L714 (16.4194, -1.8888) -> (16.4194, -2.4603)
  line L715 (16.4194, 0.5612) -> (16.4194, 1.1327)
  line L716 (16.4194, -1.312) -> (16.4194, -0.0156)
  line L717 (16.3242, -1.8888) -> (16.5147, -1.8888)
  line L718 (16.5147, -1.8888) -> (16.4194, -1.312)
  line L719 (16.3242, 0.5612) -> (16.5147, 0.5612)
  line L720 (16.5147, 0.5612) -> (16.4194, -0.0156)
  line L721 (0.6503, -14.8852) -> (0.6503, -16.8907)
  line L722 (13.6625, -14.8852) -> (13.6625, -16.8907)
  line L723 (1.2218, -16.7267) -> (13.091, -16.7267)
  line L724 (1.2218, -16.6314) -> (1.2218, -16.8219)
  line L725 (1.2218, -16.8219) -> (0.6503, -16.7267)
  line L726 (13.091, -16.6314) -> (13.091, -16.8219)
  line L727 (13.091, -16.8219) -> (13.6625, -16.7267)
  line L728 (29.802, -13.9538) -> (30.9503, -13.9538)
  line L729 (28.7755, -11.7525) -> (30.9503, -11.7525)
  line L730 (30.7863, -13.3823) -> (30.7863, -12.324)
  line L731 (30.691, -13.3823) -> (30.8815, -13.3823)
  line L732 (30.8815, -13.3823) -> (30.7863, -13.9538)
  line L733 (30.691, -12.324) -> (30.8815, -12.324)
  line L734 (30.8815, -12.324) -> (30.7863, -11.7525)
  line L735 (24.5104, -14.1179) -> (24.5104, -16.3933)
  line L736 (29.638, -14.1179) -> (29.638, -16.3933)
  line L737 (25.0872, -16.2293) -> (29.0612, -16.2293)
  line L738 (25.0872, -16.134) -> (25.0872, -16.3245)
  line L739 (25.0872, -16.3245) -> (24.5104, -16.2293)
  line L740 (29.0612, -16.134) -> (29.0612, -16.3245)
  line L741 (29.0612, -16.3245) -> (29.638, -16.2293)
  line L742 (0.2904, -14.6841) -> (0.2904, -15.8165)
  line L743 (1.0101, -14.6841) -> (1.0101, -15.8165)
  line L744 (-0.2811, -15.6525) -> (-0.8579, -15.6525)
  line L745 (1.5816, -15.6525) -> (5.4233, -15.6525)
  line L746 (0.2904, -15.6525) -> (1.0101, -15.6525)
  line L747 (-0.2811, -15.5572) -> (-0.2811, -15.7477)
  line L748 (-0.2811, -15.7477) -> (0.2904, -15.6525)
  line L749 (1.5816, -15.5572) -> (1.5816, -15.7477)
  line L750 (1.5816, -15.7477) -> (1.0101, -15.6525)
  line L751 (28.6114, -11.5885) -> (28.6114, -10.3925)
  line L752 (25.537, -11.5885) -> (25.537, -10.3925)
  line L753 (28.0399, -10.5566) -> (26.1138, -10.5566)
  line L754 (28.0399, -10.4613) -> (28.0399, -10.6518)
  line L755 (28.0399, -10.6518) -> (28.6114, -10.5566)
  line L756 (26.1138, -10.4613) -> (26.1138, -10.6518)
  line L757 (26.1138, -10.6518) -> (25.537, -10.5566)
  line L758 (14.1387, -12.2023) -> (14.1387, -10.7524)
  line L759 (14.488, -12.2023) -> (14.488, -10.7524)
  line L760 (15.0647, -10.9164) -> (15.6362, -10.9164)
  line L761 (13.5672, -10.9164) -> (9.5614, -10.9164)
  line L762 (14.488, -10.9164) -> (14.1387, -10.9164)
  line L763 (15.0647, -10.8212) -> (15.0647, -11.0117)
  line L764 (15.0647, -11.0117) -> (14.488, -10.9164)
  line L765 (13.5672, -10.8212) -> (13.5672, -11.0117)
  line L766 (13.5672, -11.0117) -> (14.1387, -10.9164)
  line L767 (15.3135, -11.7525) -> (16.6152, -11.7525)
  line L768 (14.652, -12.3663) -> (16.6152, -12.3663)
  line L769 (16.4512, -11.1757) -> (16.4512, -10.6042)
  line L770 (16.4512, -12.9378) -> (16.4512, -15.8853)
  line L771 (16.4512, -11.7525) -> (16.4512, -12.3663)
  line L772 (16.3559, -11.1757) -> (16.5464, -11.1757)
  line L773 (16.5464, -11.1757) -> (16.4512, -11.7525)
  line L774 (16.3559, -12.9378) -> (16.5464, -12.9378)
  line L775 (16.5464, -12.9378) -> (16.4512, -12.3663)
  line L776 (12.8158, -14.4989) -> (13.3079, -14.3666)
  line L777 (13.3079, -14.3666) -> (12.8846, -14.6523)
  line L778 (12.8475, -14.573) -> (11.9533, -14.9804)
  line L779 (11.9533, -14.9804) -> (11.4717, -14.9804)
  line L780 (27.3308, -14.7211) -> (27.1562, -14.7211)
  line L781 (26.9922, -14.7211) -> (26.8175, -14.7211)
  line L782 (27.4314, -14.52) -> (27.4261, -14.52)
  line L783 (26.7223, -14.52) -> (26.717, -14.52)
  line L784 (27.225, -14.52) -> (26.9287, -14.52)
  line L785 (26.8175, -14.7211) -> (26.717, -14.52)
  line L786 (26.717, -13.6998) -> (26.717, -14.0279)
  line L787 (26.717, -14.192) -> (26.717, -14.52)
  line L788 (26.7223, -14.52) -> (26.7223, -14.192)
  line L789 (26.7223, -14.0279) -> (26.7223, -13.6998)
  line L790 (26.7752, -14.573) -> (26.7752, -14.2184)
  line L791 (26.7752, -14.0544) -> (26.7752, -13.6998)
  line L792 (26.7911, -14.5941) -> (26.7911, -14.229)
  line L793 (26.7911, -14.065) -> (26.7911, -13.6998)
  line L794 (26.8599, -14.6047) -> (26.8599, -14.2343)
  line L795 (26.8599, -14.0702) -> (26.8599, -13.6998)
  line L796 (26.8705, -13.6998) -> (26.8705, -14.0491)
  line L797 (26.8705, -14.2131) -> (26.8705, -14.5677)
  line L798 (26.9287, -13.6998) -> (26.9287, -14.0279)
  line L799 (26.9287, -14.192) -> (26.9287, -14.52)
  line L800 (27.225, -14.52) -> (27.225, -14.192)
  line L801 (27.225, -14.0279) -> (27.225, -13.6998)
  line L802 (27.2779, -14.5677) -> (27.2779, -14.2131)
  line L803 (27.2779, -14.0491) -> (27.2779, -13.6998)
  line L804 (27.2885, -14.6047) -> (27.2885, -14.2343)
  line L805 (27.2885, -14.0702) -> (27.2885, -13.6998)
  line L806 (27.3626, -14.5941) -> (27.3626, -14.229)
  line L807 (27.3626, -14.065) -> (27.3626, -13.6998)
  line L808 (27.3785, -13.6998) -> (27.3785, -14.0544)
  line L809 (27.3785, -14.2184) -> (27.3785, -14.573)
  line L810 (27.4261, -13.6998) -> (27.4261, -14.0279)
  line L811 (27.4261, -14.192) -> (27.4261, -14.52)
  line L812 (27.4314, -13.6998) -> (27.4314, -14.0279)
  line L813 (27.4314, -14.192) -> (27.4314, -14.52)
  line L814 (27.4314, -14.52) -> (27.3308, -14.7211)
  line L815 (26.7752, -14.573) -> (26.7911, -14.5941)
  line L816 (27.3626, -14.5941) -> (27.3785, -14.573)
  line L817 (26.8599, -14.6047) -> (26.8599, -14.61)
  line L818 (26.8599, -14.61) -> (26.8546, -14.61)
  line L819 (26.8546, -14.61) -> (26.8546, -14.6206)
  line L820 (26.8546, -14.6206) -> (26.8493, -14.6206)
  line L821 (26.8493, -14.6206) -> (26.8493, -14.6259)
  line L822 (26.8493, -14.6259) -> (26.844, -14.6259)
  line L823 (26.844, -14.6259) -> (26.844, -14.6312)
  line L824 (26.844, -14.6312) -> (26.8281, -14.6312)
  line L825 (26.8281, -14.6312) -> (26.8281, -14.6259)
  line L826 (26.8281, -14.6259) -> (26.8175, -14.6259)
  line L827 (26.8175, -14.6259) -> (26.8175, -14.6206)
  line L828 (26.8175, -14.6206) -> (26.8123, -14.6206)
  line L829 (26.8123, -14.6206) -> (26.8017, -14.61)
  line L830 (26.8017, -14.61) -> (26.7964, -14.6047)
  line L831 (26.7964, -14.6047) -> (26.7964, -14.5994)
  line L832 (26.7964, -14.5994) -> (26.7911, -14.5994)
  line L833 (26.7911, -14.5994) -> (26.7911, -14.5941)
  line L834 (26.8599, -14.6047) -> (26.8705, -14.5677)
  line L835 (26.7752, -14.573) -> (26.7699, -14.5677)
  line L836 (26.7699, -14.5677) -> (26.7646, -14.5677)
  line L837 (26.7646, -14.5677) -> (26.7646, -14.5624)
  line L838 (26.7646, -14.5624) -> (26.7593, -14.5571)
  line L839 (26.7593, -14.5571) -> (26.7593, -14.5518)
  line L840 (26.7593, -14.5518) -> (26.754, -14.5518)
  line L841 (26.754, -14.5518) -> (26.754, -14.5465)
  line L842 (26.754, -14.5465) -> (26.7435, -14.5359)
  line L843 (26.7435, -14.5359) -> (26.7382, -14.5306)
  line L844 (26.7382, -14.5306) -> (26.7329, -14.5253)
  line L845 (26.7329, -14.5253) -> (26.7276, -14.5253)
  line L846 (26.7276, -14.5253) -> (26.7276, -14.52)
  line L847 (26.7276, -14.52) -> (26.7223, -14.52)
  line L848 (26.9287, -14.52) -> (26.9075, -14.52)
  line L849 (26.9075, -14.52) -> (26.9022, -14.5253)
  line L850 (26.9022, -14.5253) -> (26.8969, -14.5253)
  line L851 (26.8969, -14.5253) -> (26.8969, -14.5306)
  line L852 (26.8969, -14.5306) -> (26.8916, -14.5306)
  line L853 (26.8916, -14.5306) -> (26.8916, -14.5359)
  line L854 (26.8916, -14.5359) -> (26.8863, -14.5359)
  line L855 (26.8863, -14.5359) -> (26.8863, -14.5412)
  line L856 (26.8863, -14.5412) -> (26.881, -14.5412)
  line L857 (26.881, -14.5412) -> (26.881, -14.5465)
  line L858 (26.881, -14.5465) -> (26.8758, -14.5518)
  line L859 (26.8758, -14.5518) -> (26.8758, -14.5624)
  line L860 (26.8758, -14.5624) -> (26.8705, -14.5624)
  line L861 (26.8705, -14.5624) -> (26.8705, -14.5677)
  line L862 (27.3626, -14.5941) -> (27.3573, -14.5941)
  line L863 (27.3573, -14.5941) -> (27.3573, -14.5994)
  line L864 (27.3573, -14.5994) -> (27.352, -14.6047)
  line L865 (27.352, -14.6047) -> (27.3467, -14.61)
  line L866 (27.3467, -14.61) -> (27.3361, -14.6206)
  line L867 (27.3361, -14.6206) -> (27.3308, -14.6206)
  line L868 (27.3308, -14.6206) -> (27.3308, -14.6259)
  line L869 (27.3308, -14.6259) -> (27.3255, -14.6259)
  line L870 (27.3255, -14.6259) -> (27.3203, -14.6312)
  line L871 (27.3203, -14.6312) -> (27.3044, -14.6312)
  line L872 (27.3044, -14.6312) -> (27.3044, -14.6259)
  line L873 (27.3044, -14.6259) -> (27.2991, -14.6259)
  line L874 (27.2991, -14.6259) -> (27.2991, -14.6206)
  line L875 (27.2991, -14.6206) -> (27.2938, -14.6206)
  line L876 (27.2938, -14.6206) -> (27.2938, -14.61)
  line L877 (27.2938, -14.61) -> (27.2885, -14.6047)
  line L878 (27.4261, -14.52) -> (27.4208, -14.52)
  line L879 (27.4208, -14.52) -> (27.4208, -14.5253)
  line L880 (27.4208, -14.5253) -> (27.4155, -14.5253)
  line L881 (27.4155, -14.5253) -> (27.4102, -14.5306)
  line L882 (27.4102, -14.5306) -> (27.4049, -14.5359)
  line L883 (27.4049, -14.5359) -> (27.4049, -14.5412)
  line L884 (27.4049, -14.5412) -> (27.3996, -14.5412)
  line L885 (27.3996, -14.5412) -> (27.3943, -14.5465)
  line L886 (27.3943, -14.5465) -> (27.3943, -14.5518)
  line L887 (27.3943, -14.5518) -> (27.389, -14.5518)
  line L888 (27.389, -14.5518) -> (27.389, -14.5571)
  line L889 (27.389, -14.5571) -> (27.3838, -14.5624)
  line L890 (27.3838, -14.5624) -> (27.3838, -14.5677)
  line L891 (27.3838, -14.5677) -> (27.3785, -14.5677)
  line L892 (27.3785, -14.5677) -> (27.3785, -14.573)
  line L893 (27.2885, -14.6047) -> (27.2779, -14.5677)
  line L894 (27.2779, -14.5677) -> (27.2779, -14.5624)
  line L895 (27.2779, -14.5624) -> (27.2726, -14.5571)
  line L896 (27.2726, -14.5571) -> (27.2726, -14.5518)
  line L897 (27.2726, -14.5518) -> (27.2673, -14.5465)
  line L898 (27.2673, -14.5465) -> (27.2673, -14.5412)
  line L899 (27.2673, -14.5412) -> (27.262, -14.5412)
  line L900 (27.262, -14.5412) -> (27.262, -14.5359)
  line L901 (27.262, -14.5359) -> (27.2568, -14.5306)
  line L902 (27.2568, -14.5306) -> (27.2515, -14.5253)
  line L903 (27.2515, -14.5253) -> (27.2462, -14.5253)
  line L904 (27.2462, -14.5253) -> (27.2462, -14.52)
  line L905 (27.2462, -14.52) -> (27.225, -14.52)
  line L906 (0.2904, -13.8004) -> (0.2904, -14.0755)
  line L907 (0.2904, -14.2396) -> (0.2904, -14.52)
  line L908 (0.3222, -14.52) -> (0.3222, -14.2396)
  line L909 (0.3222, -14.0755) -> (0.3222, -13.8004)
  line L910 (0.3857, -14.5677) -> (0.3857, -14.266)
  line L911 (0.3857, -14.102) -> (0.3857, -13.8004)
  line L912 (0.4227, -14.6047) -> (0.4227, -14.2872)
  line L913 (0.4227, -14.1232) -> (0.4227, -13.8004)
  line L914 (0.5074, -14.5941) -> (0.5074, -14.2766)
  line L915 (0.5074, -14.1179) -> (0.5074, -13.8004)
  line L916 (0.5127, -13.8004) -> (0.5127, -14.1073)
  line L917 (0.5127, -14.266) -> (0.5127, -14.573)
  line L918 (0.7138, -14.52) -> (0.7138, -14.2396)
  line L919 (0.7138, -14.0755) -> (0.7138, -13.8004)
  line L920 (0.3963, -14.7211) -> (0.2904, -14.52)
  line L921 (0.7878, -14.573) -> (0.7931, -14.5835)
  line L922 (0.7931, -14.5835) -> (0.7931, -14.5941)
  line L923 (0.7878, -14.573) -> (0.7878, -14.266)
  line L924 (0.7878, -14.1073) -> (0.7878, -13.8004)
  line L925 (0.7931, -14.5941) -> (0.7931, -14.2766)
  line L926 (0.7931, -14.1179) -> (0.7931, -13.8004)
  line L927 (0.8778, -14.6047) -> (0.8778, -14.2872)
  line L928 (0.8778, -14.1232) -> (0.8778, -13.8004)
  line L929 (0.9148, -13.8004) -> (0.9148, -14.102)
  line L930 (0.9148, -14.266) -> (0.9148, -14.5677)
  line L931 (0.9783, -13.8004) -> (0.9783, -14.0755)
  line L932 (0.9783, -14.2396) -> (0.9783, -14.52)
  line L933 (1.0101, -13.8004) -> (1.0101, -14.0755)
  line L934 (1.0101, -14.2396) -> (1.0101, -14.52)
  line L935 (0.3857, -14.5677) -> (0.3645, -14.5465)
  line L936 (0.3645, -14.5465) -> (0.3486, -14.5306)
  line L937 (0.3486, -14.5306) -> (0.3327, -14.52)
  line L938 (0.3327, -14.52) -> (0.3222, -14.52)
  line L939 (0.3857, -14.5677) -> (0.4015, -14.5888)
  line L940 (0.4015, -14.5888) -> (0.4227, -14.6047)
  line L941 (0.7878, -14.573) -> (0.772, -14.5518)
  line L942 (0.772, -14.5518) -> (0.7561, -14.5306)
  line L943 (0.7561, -14.5306) -> (0.7349, -14.52)
  line L944 (0.7349, -14.52) -> (0.7138, -14.52)
  line L945 (0.5074, -14.5941) -> (0.5127, -14.5835)